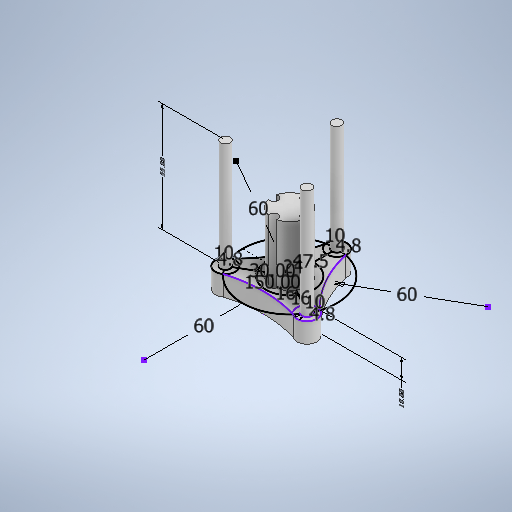
# Autodesk Inventor part: wheel_connection.0001
Saved by Autodesk Inventor 2025.1 (Build 291241000, 241)
## iProperties
Created: 2024-10-11
Part Number: wheel_connection.0001
Material: 일반
Document SubType Name: Sheet Metal
Designer: goode
Density: 1 g/cm^3
Sheet Metal Rule: 기본값_mm
Appearance: 기본값
Author: goode
Autodesk Inventor part; units mm, degrees
ref_plane "YZ Plane" through (0, 0, 0) normal (1, 0, 0) x (0, 1, 0)
ref_plane "XZ Plane" through (0, 0, 0) normal (0, 1, 0) x (-1, 0, 0)
ref_plane "XY Plane" through (0, 0, 0) normal (0, 0, 1) x (1, 0, 0)
sketch "스케치1" plane through (0, 0, 0) normal (0, 1, 0) x (-1, 0, 0)
  circle A0 centre (0, 0) radius 23.75
  circle A1 centre (0, -23.75) radius 2.4
  line L0 (0, 0) -> (0, -23.75)
  line L1 (0, 0) -> (20.5681, 11.875)
  line L2 (0, 0) -> (23.75, 0) construction
  line L3 (0, 0) -> (-20.5681, 11.875)
  line L4 (0, 0) -> (23.75, 0) construction
  circle A2 centre (20.5681, 11.875) radius 2.4
  circle A3 centre (-20.5681, 11.875) radius 2.4
  circle A4 centre (20.5681, 11.875) radius 5
  circle A5 centre (-20.5681, 11.875) radius 5
  circle A6 centre (0, -23.75) radius 5
  circle A7 centre (0, 0) radius 12
  arc A8 (-17.6262, 15.9179) -> (17.6262, 15.9179) centre (0, 73.2705) ccw
  arc A9 (22.5984, 7.3058) -> (4.9722, -23.2237) centre (63.4541, -36.6352) ccw
  arc A10 (-4.9722, -23.2237) -> (-22.5984, 7.3058) centre (-63.4541, -36.6352) ccw
  point P0 (-4.9722, -23.2237)
  dimension "d0" = 47.5
  dimension "d8" = 10
  dimension "d1" = 4.8
  dimension "d2" = 30
  dimension "d3" = 150
  dimension "d4" = 4.8
  dimension "d5" = 4.8
  dimension "d6" = 10
  dimension "d7" = 10
  dimension "d9" = 24
  dimension "d10" = 60
  dimension "d11" = 60
  dimension "d12" = 60
  constraints: 10 end point, 10 point on circle, 9 centre point, 6 coincident, 2 equal length, 2 horizontal, 1 vertical, 15 other
  measures "d1" diameter of A1
  measures "d2" angle of L2 L1
  measures "d3" angle of L4 L3
  measures "d4" diameter of A2
  measures "d5" diameter of A3
  measures "d6" diameter of A4
  measures "d7" diameter of A5
  measures "d9" diameter of A7
  measures "d10" radius of A8
  measures "d11" radius of A9
  measures "d12" radius of A10
sketch "스케치2" plane through (0, 0, 0) normal (0, 1, 0) x (-1, 0, 0)
  point P0 (0, 0)
extrude "돌출3" add sketch "스케치1" against normal blind 5 contours A4 L1 A2 A0 | A0 A2 A4 | A9 A6 L0 A7 L1 A4 | A6 A0 A1 | A0 A1 L0 A6 | A2 L1 A0 | A0 A2 | A4 A0 A2 L1 | L1 A7 L3 A5 A8 A4 | A1 A0 | A0 L0 A1 | A6 A10 A5 L3 A7 L0 | L0 A1 A0 A6 | L1 A2 A0 | A7 L0 L1 | L1 L3 A7 | A0 A1 L0 | A7 L3 L0 | A5 L3 A3 A0 | A0 A3 A5 | A0 A3 L3 A5 | A3 L3 A0 | A0 A3 | A0 L3 A3
sketch "스케치3" plane through (0, -5, 0) normal (0, -1, 0) x (1, 0, 0)
  point P0 (0, 0)
extrude "돌출4" add sketch "스케치1" against normal blind 10 contours A4 L1 A2 A0 | A0 A2 A4 | A9 A6 L0 A7 L1 A4 | A6 A0 A1 | A0 A1 L0 A6 | A2 L1 A0 | A0 A2 | A4 A0 A2 L1 | L1 A7 L3 A5 A8 A4 | A1 A0 | A0 L0 A1 | A6 A10 A5 L3 A7 L0 | L0 A1 A0 A6 | L1 A2 A0 | A7 L0 L1 | L1 L3 A7 | A0 A1 L0 | A7 L3 L0 | A5 L3 A3 A0 | A0 A3 A5 | A0 A3 L3 A5 | A3 L3 A0 | A0 A3 | A0 L3 A3
extrude "돌출5" add sketch "스케치1" along normal blind 55 contours A2 L1 A0 | A0 A2 | A1 A0 | A0 L0 A1 | L1 A2 A0 | A0 A1 L0 | A3 L3 A0 | A0 A3 | A0 L3 A3
sketch "스케치4" plane through (0, -10, 0) normal (0, -1, 0) x (1, 0, 0)
  circle A0 centre (0, 0) radius 8
  circle A1 centre (0, 0) radius 8
  point P0 (8, 0)
  point P1 (0, -8)
  point P2 (0, 8)
  point P3 (-8, 0)
  point P4 (-8, 0)
  point P5 (-8, 0)
  point P6 (0, 8)
  point P7 (8, 0)
  point P8 (0, -8)
  dimension "d24" = 16
  dimension "d26" = 16
  constraints: 7 point on circle, 4 coincident, 2 centre point
  measures "d24" diameter of A0
  measures "d26" diameter of A1
sketch "스케치5" plane through (0, 0, 0) normal (0, 1, 0) x (1, 0, 0)
  circle A0 centre (0, 0) radius 8
  point P0 (8, 0)
  point P1 (0, -8)
  point P2 (-8, 0)
  point P3 (0, 8)
  dimension "d27" = 16
  constraints: 4 point on circle, 1 centre point, 1 coincident
  measures "d27" diameter of A0
hole "구멍1" at (0, 0, 8) at (-8, 0, 0) at (0, 0, -8) at (8, 0, 0) direction (0, -1, 0) diameter 2.2 end through all counterbore diameter 4.2 counterbore depth 7
sketch "스케치6" plane through (0, 0, 0) normal (0, 1, 0) x (1, 0, 0)
  point P0 (0, 0)
sketch "스케치7" plane through (0, 0, 0) normal (0, 1, 0) x (1, 0, 0)
  circle A0 centre (0, 0) radius 8.95
  circle A1 centre (0, 0) radius 8
  circle A2 centre (0, 8) radius 2.1
  circle A3 centre (-8, 0) radius 2.1
  circle A4 centre (0, -8) radius 2.1
  circle A5 centre (8, 0) radius 2.1
  point P0 (8.7308, 1.9687)
  point P1 (1.9687, 8.7308)
  point P2 (-1.9687, 8.7308)
  point P3 (-8.7308, 1.9687)
  point P4 (-8.7308, -1.9687)
  point P5 (-1.9687, -8.7308)
  point P6 (1.9687, -8.7308)
  point P7 (8.7308, -1.9687)
  dimension "d37" = 16
  dimension "d36" = 17.9
  dimension "d38" = 4.2
  dimension "d41" = 360
  constraints: 5 centre point, 2 coincident, 1 vertical alignment, 11 other
  measures "d36" diameter of A0
  measures "d38" diameter of A2
extrude "돌출6" add sketch "스케치7" along normal blind 30 contours A5 A1 A2 A0 | A0 A4 A1 A5 | A5 A1 A4 A3 A2 | A2 A1 A3 A0 | A0 A3 A1 A4
equation "\"d19\" = d7"
equation "\"TransitionRadius\" = BendRadius"
equation "\"BendRadius\" = 0.5"
